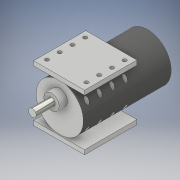
# Autodesk Inventor part: Big Motor
Saved by Autodesk Inventor 2019 (Build 230136000, 136)
## iProperties
Created: 2019-01-28
Part Number: Big Motor
Material: Generic
Document SubType Name: Modeling
Designer: scigu
Density: 1 g/cm^3
Appearance: Default
Author: scigu
Autodesk Inventor part; units mm, degrees
ref_plane "YZ Plane" through (0, 0, 0) normal (1, 0, 0) x (0, 1, 0)
ref_plane "XY Plane" through (0, 0, 0) normal (0, 0, 1) x (1, 0, 0)
sketch "Sketch1" plane through (0, 0, 0) normal (0, 0, 1) x (1, 0, 0)
  circle A0 centre (0, 0) radius 18.5
  dimension "d0" = 37
  constraints: 1 centre point, 1 coincident
  measures "d0" diameter of A0
extrude "Extrusion1" add sketch "Sketch1" along normal blind 69
sketch "Sketch2" plane through (0, 0, 69) normal (0, 0, 1) x (1, 0, 0)
  line L0 (0, 0) -> (0, 12) construction
  line L1 (0, 0) -> (0, 18.5) construction
  line L2 (0, 18.5) -> (0, 1.1) construction
  line L3 (0, 1.1) -> (0, 7.1) construction
  circle A0 centre (0, 7.1) radius 6
  dimension "d5" = 18.5
  dimension "d6" = 17.4
  dimension "d7" = 6
  constraints: 8 end point, 2 point on line, 2 vertical, 1 coincident, 1 vertical alignment, 2 other
  measures "d5" distance of L0.start L1.end
  measures "d6" distance of L1.end L2.end
  measures "d7" distance of L2.end L3.end
extrude "Extrusion2" add sketch "Sketch2" along normal blind 6.5
sketch "Sketch3" plane through (0, 7.1, 75.5) normal (0, 0, 1) x (1, 0, 0)
  circle A0 centre (0, 0) radius 3
  point P0 (0, -7.1)
  dimension "d10" = 6
  constraints: 1 centre point
  measures "d10" diameter of A0
extrude "Extrusion3" add sketch "Sketch3" along normal blind 15
ref_plane "Work Plane1" through (0, 18.5, 0) normal (0, 1, 0) x (-1, 0, 0)
sketch "Sketch4" plane through (0, 18.5, 0) normal (0, 1, 0) x (-1, 0, 0)
  line L0 (0, 0) -> (0, 69.5) construction
  line L1 (0, 69.5) -> (-20, 69.5) construction
  line L2 (-20, 69.5) -> (-20, 28.5) construction
  line L3 (-20, 28.5) -> (0, 28.5) construction
  line L4 (0, 28.5) -> (0, 69.5) construction
  line L5 (-20, 69.5) -> (20, 69.5)
  line L6 (20, 69.5) -> (20, 28.5)
  line L7 (20, 28.5) -> (-20, 28.5)
  line L8 (-20, 28.5) -> (-20, 69.5)
  dimension "d13" = 69.5
  dimension "d14" = 20
  dimension "d15" = 41
  dimension "d16" = 40
  dimension "d17" = 41
  constraints: 18 end point, 4 parallel, 2 horizontal, 2 perpendicular, 1 vertical
  measures "d13" distance of L0.start L0.end
  measures "d14" distance of L3.end L2.end
  measures "d15" distance of L2.end L1.end
  measures "d16" distance of L6.end L7.end
  measures "d17" distance of L5.end L6.end
extrude "Extrusion4" add sketch "Sketch4" along normal blind 3.5
sketch "Sketch5" plane through (0, 22, 0) normal (0, 1, 0) x (1, 0, 0)
  line L0 (20, -69.5) -> (-20, -69.5) construction
  line L1 (-20, -69.5) -> (-15.5, -69.5) construction
  line L2 (-15.5, -69.5) -> (-15.5, -63.5) construction
  line L3 (-15.5, -63.5) -> (-20, -63.5) construction
  line L4 (-20, -63.5) -> (-20, -69.5) construction
  line L5 (-15.5, -63.5) -> (-15.5, -53.5) construction
  line L6 (-15.5, -63.5) -> (-5.5, -63.5) construction
  line L7 (20, -69.5) -> (15.5, -69.5) construction
  line L8 (15.5, -69.5) -> (15.5, -63.5) construction
  line L9 (15.5, -63.5) -> (20, -63.5) construction
  line L10 (20, -63.5) -> (20, -69.5) construction
  point P0 (0, 0)
  dimension "d20" = 4.5
  dimension "d21" = 6
  dimension "d22" = 10
  dimension "d23" = 90
  dimension "d24" = 4.5
  dimension "d25" = 6
  constraints: 20 end point, 4 parallel, 3 horizontal, 3 perpendicular, 2 coincident, 1 vertical
  measures "d20" distance of L3.end L2.end
  measures "d21" distance of L2.end L1.end
  measures "d22" distance of L2.end L5.end
  measures "d23" angle of L6 L5
  measures "d24" distance of L8.end L9.end
  measures "d25" distance of L7.end L8.end
hole "Hole1" at (-15.5, 22, 63.5) at (15.5, 22, 63.5) direction (0, -1, 0) diameter 3 end through all
pattern_linear "Rectangular Pattern1" count 4 spacing 10 along (0, 0, -1) of "Hole1"
mirror "Mirror1" about plane through (0, 0, 0) normal (0, 1, 0) of "Extrusion4"
body "Solid1"
